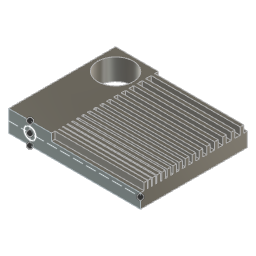
gapTestv4 (Autodesk Fusion 360 design; units mm, degrees)
Autodesk Fusion 360 part; units mm, degrees
sketch "Sketch1" plane through (0, 0, 0) normal (0, 0, 1) x (1, 0, 0)
  line L0 (0, 0) -> (37, 0)
  line L1 (37, 0) -> (37, 30)
  line L2 (37, 30) -> (0, 30)
  line L3 (0, 30) -> (0, 0)
  line L4 (12, 30) -> (12, 0) construction
  line L5 (12, 1) -> (37, 1)
  line L6 (12, 2) -> (37, 2)
  line L7 (12, 2.1) -> (37, 2.1)
  line L8 (12, 3.1) -> (37, 3.1)
  line L9 (12, 3.3) -> (37, 3.3)
  line L10 (12, 4.3) -> (37, 4.3)
  line L11 (12, 4.6) -> (37, 4.6)
  line L12 (12, 5.6) -> (37, 5.6)
  line L13 (12, 6) -> (37, 6)
  line L14 (12, 7) -> (37, 7)
  line L15 (12, 7.5) -> (37, 7.5)
  line L16 (12, 8.5) -> (37, 8.5)
  line L17 (12, 9.1) -> (37, 9.1)
  line L18 (12, 10.1) -> (37, 10.1)
  line L19 (12, 10.8) -> (37, 10.8)
  line L20 (37, 11.8) -> (12, 11.8)
  line L21 (12, 12.6) -> (37, 12.6)
  line L22 (37, 13.6) -> (12, 13.6)
  line L23 (12, 14.5) -> (37, 14.5)
  line L24 (37, 15.5) -> (12, 15.5)
  line L25 (12, 16.5) -> (37, 16.5)
  line L26 (37, 17.5) -> (12, 17.5)
  line L27 (12, 18.6) -> (37, 18.6)
  line L28 (37, 19.6) -> (12, 19.6)
  line L29 (12, 23.1) -> (37, 23.1)
  line L30 (12, 20.8) -> (37, 20.8)
  line L31 (12, 21.8) -> (37, 21.8)
  line L32 (12, 24.1) -> (37, 24.1)
  line L33 (37, 25.5) -> (12, 25.5)
  line L34 (12, 26.5) -> (37, 26.5)
  line L35 (37, 28) -> (12, 28)
  line L36 (12, 29) -> (37, 29)
  line L37 (12, 30) -> (12, 0)
  circle A0 centre (6, 24) radius 5
  dimension "d4" = 30
  dimension "d5" = 37
  dimension "d6" = 25
  dimension "d11" = 1
  dimension "d12" = 1
  dimension "d13" = 0.1
  dimension "d14" = 1
  dimension "d15" = 0.2
  dimension "d16" = 1
  dimension "d17" = 0.3
  dimension "d18" = 1
  dimension "d19" = 0.4
  dimension "d20" = 1
  dimension "d21" = 0.5
  dimension "d22" = 1
  dimension "d23" = 0.6
  dimension "d24" = 1
  dimension "d25" = 0.7
  dimension "d26" = 1
  dimension "d27" = 0.8
  dimension "d28" = 1
  dimension "d29" = 0.9
  dimension "d30" = 1
  dimension "d31" = 1
  dimension "d32" = 1
  dimension "d33" = 1.1
  dimension "d34" = 1
  dimension "d35" = 1.2
  dimension "d36" = 1
  dimension "d37" = 1.3
  dimension "d38" = 1
  dimension "d39" = 1.4
  dimension "d40" = 1
  dimension "d41" = 1.5
  dimension "d42" = 1
  dimension "d47" = 10
  constraint horizontal L0
  constraint vertical L1
  constraint horizontal L2
  constraint vertical L3
  constraint coincident L0.start L3.end
  constraint coincident L2 L4.start
  constraint coincident L0 L4.end
  constraint perpendicular L0 L4
  constraint coincident L4 L5.start
  constraint coincident L1 L5.end
  constraint perpendicular L1 L5
  constraint coincident L4 L6.start
  constraint coincident L1 L6.end
  constraint perpendicular L1 L6
  constraint coincident L4 L7.start
  constraint coincident L1 L7.end
  constraint perpendicular L1 L7
  constraint coincident L4 L8.start
  constraint coincident L1 L8.end
  constraint perpendicular L1 L8
  constraint coincident L4 L9.start
  constraint coincident L1 L9.end
  constraint perpendicular L1 L9
  constraint coincident L4 L10.start
  constraint coincident L1 L10.end
  constraint perpendicular L1 L10
  constraint coincident L4 L11.start
  constraint coincident L1 L11.end
  constraint perpendicular L1 L11
  constraint coincident L4 L12.start
  constraint coincident L1 L12.end
  constraint perpendicular L1 L12
  constraint coincident L4 L13.start
  constraint coincident L1 L13.end
  constraint perpendicular L1 L13
  constraint coincident L4 L14.start
  constraint coincident L1 L14.end
  constraint perpendicular L1 L14
  constraint coincident L4 L15.start
  constraint coincident L1 L15.end
  constraint perpendicular L1 L15
  constraint coincident L4 L16.start
  constraint coincident L1 L16.end
  constraint perpendicular L1 L16
  constraint coincident L4 L17.start
  constraint coincident L1 L17.end
  constraint perpendicular L1 L17
  constraint coincident L4 L18.start
  constraint coincident L1 L18.end
  constraint perpendicular L1 L18
  constraint coincident L4 L19.start
  constraint coincident L1 L19.end
  constraint perpendicular L1 L19
  constraint coincident L1 L20.start
  constraint coincident L4 L20.end
  constraint perpendicular L4 L20
  constraint coincident L4 L21.start
  constraint coincident L1 L21.end
  constraint perpendicular L1 L21
  constraint coincident L1 L22.start
  constraint coincident L4 L22.end
  constraint perpendicular L4 L22
  constraint coincident L4 L23.start
  constraint coincident L1 L23.end
  constraint perpendicular L1 L23
  constraint coincident L1 L24.start
  constraint coincident L4 L24.end
  constraint perpendicular L4 L24
  constraint coincident L4 L25.start
  constraint coincident L1 L25.end
  constraint perpendicular L1 L25
  constraint coincident L1 L26.start
  constraint coincident L4 L26.end
  constraint perpendicular L4 L26
  constraint coincident L4 L27.start
  constraint coincident L1 L27.end
  constraint perpendicular L1 L27
  constraint coincident L1 L28.start
  constraint coincident L4 L28.end
  constraint perpendicular L4 L28
  constraint coincident L4 L29.start
  constraint coincident L1 L29.end
  constraint perpendicular L1 L29
  constraint coincident L4 L30.start
  constraint coincident L1 L30.end
  constraint perpendicular L1 L30
  constraint coincident L4 L31.start
  constraint coincident L1 L31.end
  constraint perpendicular L1 L31
  constraint coincident L4 L32.start
  constraint coincident L1 L32.end
  constraint perpendicular L1 L32
  constraint coincident L1 L33.start
  constraint coincident L4 L33.end
  constraint perpendicular L4 L33
  constraint coincident L4 L34.start
  constraint coincident L1 L34.end
  constraint perpendicular L1 L34
  constraint coincident L1 L35.start
  constraint coincident L4 L35.end
  constraint perpendicular L4 L35
  constraint coincident L4 L36.start
  constraint coincident L1 L36.end
  constraint perpendicular L1 L36
  constraint perpendicular L0 L37
  constraint coincident L4.start L37.start
  measures "d4" distance of L0.start L2.end
  measures "d5" distance of L1 L3
  measures "d6" distance of L1 L4
  measures "d11" distance of L0 L5
  measures "d12" distance of L5 L6
  measures "d13" distance of L6 L7
  measures "d14" distance of L7 L8
  measures "d15" distance of L8 L9
  measures "d16" distance of L9 L10
  measures "d17" distance of L10 L11
  measures "d18" distance of L11 L12
  measures "d19" distance of L12 L13
  measures "d20" distance of L13 L14
  measures "d21" distance of L14 L15
  measures "d22" distance of L15 L16
  measures "d23" distance of L16 L17
  measures "d24" distance of L17 L18
  measures "d25" distance of L18 L19
  measures "d26" distance of L19 L20
  measures "d27" distance of L20 L21
  measures "d28" distance of L21 L22
  measures "d29" distance of L22 L23
  measures "d30" distance of L23 L24
  measures "d31" distance of L24 L25
  measures "d32" distance of L25 L26
  measures "d33" distance of L26 L27
  measures "d34" distance of L27 L28
  measures "d35" distance of L28 L30
  measures "d36" distance of L30 L31
  measures "d37" distance of L29 L31
  measures "d38" distance of L29 L32
  measures "d39" distance of L32 L33
  measures "d40" distance of L33 L34
  measures "d41" distance of L34 L35
  measures "d42" distance of L35 L36
  measures "d47" diameter of A0
extrude "Extrude5" add sketch "Sketch1" along normal blind 6 contours L0 L2 L3 L37
extrude "Extrude6" add sketch "Sketch1" along normal blind 6 contours L1 L5 L6 L37 | L1 L35 L36 L37 | L1 L7 L8 L37 | L1 L33 L34 L37 | L1 L9 L10 L37 | L1 L29 L32 L37 | L1 L11 L12 L37 | L1 L30 L31 L37 | L1 L13 L14 L37 | L1 L27 L28 L37 | L1 L15 L16 L37 | L1 L25 L26 L37 | L1 L17 L18 L37 | L1 L23 L24 L37 | L1 L19 L20 L37 | L1 L21 L22 L37
extrude "Extrude7" add sketch "Sketch1" along normal blind 4 contours L0 L1 L5 L37 | L1 L2 L36 L37 | L1 L6 L7 L37 | L1 L34 L35 L37 | L1 L8 L9 L37 | L1 L32 L33 L37 | L1 L10 L11 L37 | L1 L29 L31 L37 | L1 L12 L13 L37 | L1 L28 L30 L37 | L1 L14 L15 L37 | L1 L26 L27 L37 | L1 L16 L17 L37 | L1 L24 L25 L37 | L1 L18 L19 L37 | L1 L22 L23 L37 | L1 L20 L21 L37
sketch "Sketch3" plane through (0, 0, 0) normal (0, -1, 0) x (1, 0, 0)
  line L0 (0, 0) -> (37, 0)
  line L1 (37, 0) -> (37, 4)
  line L2 (37, 4) -> (12, 4)
  line L3 (12, 4) -> (12, 6)
  line L4 (12, 6) -> (0, 6)
  line L5 (0, 6) -> (0, 0)
  line L6 (0, 3) -> (37, 3) construction
  line L7 (6, 0) -> (6, 6) construction
  circle A0 centre (6, 3) radius 1.6
  dimension "d60" = 6
  dimension "d61" = 3.2
  constraint midpoint L5 L6.start
  constraint coincident L1 L6.end
  constraint perpendicular L1 L6
  constraint coincident L0 L7.start
  constraint coincident L4 L7.end
  constraint perpendicular L4 L7
  constraint midpoint L7 A0.centre
  measures "d60" distance of L5 L7
  measures "d61" diameter of A0
extrude "Extrude8" [suppressed]
thread "Thread2" [suppressed]
equation "length = 37 mm"
equation "width = 30 mm"
equation "thickness = 6 mm"
equation "d4 = width"
equation "d5 = length"
equation "d6 = comb_length"
equation "comb_length = 25 mm"
equation "comb_height = 2 mm"
equation "comb_width = 1 mm"
equation "comb_spacing = 0.1 mm"
equation "d12 = comb_width"
equation "d13 = comb_spacing"
equation "d14 = comb_width"
equation "d15 = comb_spacing * 2"
equation "d16 = comb_width"
equation "d17 = comb_spacing * 3"
equation "d18 = comb_width"
equation "d19 = comb_spacing * 4"
equation "d20 = comb_width"
equation "d21 = comb_spacing * 5"
equation "d22 = comb_width"
equation "d23 = comb_spacing * 6"
equation "d24 = comb_width"
equation "d25 = comb_spacing * 7"
equation "d26 = comb_width"
equation "d27 = comb_spacing * 8"
equation "d28 = comb_width"
equation "d29 = comb_spacing * 9"
equation "d30 = comb_width"
equation "d31 = comb_spacing * 10"
equation "d32 = comb_width"
equation "d33 = comb_spacing * 11"
equation "d34 = comb_width"
equation "d35 = comb_spacing * 12"
equation "d36 = comb_width"
equation "d37 = comb_spacing * 13"
equation "d38 = comb_width"
equation "d39 = comb_spacing * 14"
equation "d40 = comb_width"
equation "d41 = comb_spacing * 15"
equation "d42 = comb_width"
equation "d54 = thickness"
equation "d56 = thickness"
equation "d58 = thickness - comb_height"
equation "d62 = -width"
